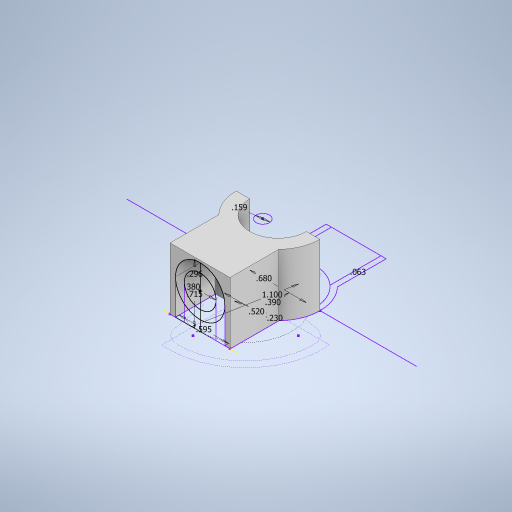
# Autodesk Inventor part: Ball Valve Mount
Saved by Autodesk Inventor 2023 (Build 270158000, 158)
## iProperties
Created: 2023-02-08
Part Number: Ball Valve Mount
Material: Generic
Document SubType Name: Modeling
Designer: tommy
Density: 1 g/cm^3
Appearance: Default
Author: tommy
Autodesk Inventor part; units mm, degrees
ref_plane "YZ Plane" through (0, 0, 0) normal (1, 0, 0) x (0, 1, 0)
ref_plane "XZ Plane" through (0, 0, 0) normal (0, 1, 0) x (-1, 0, 0)
ref_plane "XY Plane" through (0, 0, 0) normal (0, 0, 1) x (1, 0, 0)
sketch "Sketch1" plane through (0, 0, 0) normal (0, 1, 0) x (-1, 0, 0)
  circle A0 centre (0, 0) radius 8.636
  line L0 (7.5565, 23.7871) -> (-7.5565, 23.7871)
  line L1 (7.5565, -23.7871) -> (-7.5565, -23.7871)
  line L2 (7.5565, 23.7871) -> (7.5565, 8.2342)
  line L3 (7.5565, -8.2342) -> (7.5565, -23.7871)
  arc A1 (7.5565, -8.2342) -> (7.5565, 8.2342) centre (0, 0) ccw
  arc A2 (-7.5565, 8.2342) -> (-7.5565, -8.2342) centre (0, 0) ccw
  line L4 (-7.5565, -23.7871) -> (-7.5565, -8.2342)
  line L5 (-7.5565, 8.2342) -> (-7.5565, 23.7871)
  line L6 (-9.144, -8.9047) -> (-9.144, -23.7871)
  line L7 (9.144, -23.7871) -> (9.144, -8.9047)
  arc A3 (9.144, -8.9047) -> (9.144, 8.9047) centre (0, 0) ccw
  line L8 (9.144, 8.9047) -> (9.144, 23.7871)
  line L9 (-9.144, 23.7871) -> (-9.144, 8.9047)
  arc A4 (-9.144, 8.9047) -> (-9.144, -8.9047) centre (0, 0) ccw
  line L10 (7.5565, -23.7871) -> (9.144, -23.7871)
  line L11 (9.144, -23.7871) -> (-9.144, -23.7871)
  line L12 (-7.5565, 23.7871) -> (-9.144, 23.7871)
  line L13 (-9.144, 23.7871) -> (9.144, 23.7871)
  circle A5 centre (0, 0) radius 11.176
  line L14 (46.1577, 0) -> (-42.2099, 0)
  circle A6 centre (20.2123, -15.5184) radius 2.0193
  circle A7 centre (0, 9.906) radius 2.921 construction
  circle A8 centre (0, 9.906) radius 6.604 construction
  line L15 (-6.3706, 3.5354) -> (-16.823, 5.2035) construction
  arc A9 (2.286, 33.1684) -> (-23.2624, 7.62) centre (0, 9.906) ccw construction
  line L16 (4.7025, 26.729) -> (6.3706, 16.2766) construction
  arc A10 (-20.8345, 9.906) -> (-16.823, 5.2035) centre (-16.0725, 9.906) ccw construction
  line L17 (-4.7025, -6.917) -> (-6.3706, 3.5354) construction
  arc A11 (-4.7025, -6.917) -> (0, -10.9285) centre (0, -6.1665) ccw construction
  arc A12 (4.7025, 26.729) -> (0, 30.7405) centre (0, 25.9785) ccw construction
  line L18 (6.3706, 16.2766) -> (16.823, 14.6085) construction
  arc A13 (20.8345, 9.906) -> (16.823, 14.6085) centre (16.0725, 9.906) ccw construction
  arc A14 (0, 30.7405) -> (-20.8345, 9.906) centre (0, 9.906) ccw construction
  arc A15 (0, -10.9285) -> (20.8345, 9.906) centre (0, 9.906) ccw construction
  line L19 (0, 0) -> (0, 9.906)
  line L20 (2.286, 33.2805) -> (2.286, 7.62) construction
  line L21 (2.286, 7.62) -> (-23.3745, 7.62) construction
  circle A16 centre (0, 9.906) radius 13.97 construction
  point P0 (-7.5565, -8.2342)
  point P1 (-7.5565, 8.2342)
  point P2 (-12.7635, 0)
  point P3 (-8.636, 0)
  point P4 (8.636, 0)
  point P5 (12.7635, 0)
  point P6 (-12.7635, 0)
  dimension "d0" = 17.272
  dimension "d6" = 15.113
  dimension "d7" = 1.5875
  dimension "d27" = 4.0386
  dimension "d31" = 5.842
  dimension "d32" = 13.208
  dimension "d35" = 9.906
  dimension "d37" = 27.94
  constraints: 44 end point, 23 point on circle, 17 centre point, 5 coincident, 5 perpendicular, 5 point on line, 3 vertical, 2 horizontal, 1 concentric
  measures "d0" diameter of A0
  measures "d6" distance of L0.start L0.end
  measures "d7" distance between parallel lines of L4 L6
  measures "d27" diameter of A6
  measures "d31" diameter of A7
  measures "d32" diameter of A8
  measures "d35" distance of L19.start L19.end
  measures "d37" diameter of A16
extrude "Extrusion1" add sketch "Sketch1" along normal blind 18.796 contours A0 L14 A2 A5 A1 | A1 L2 L13 L8 A3 L14 | L14 A4 L9 L12 L5 A2 | A5 L5 L0 L2 picked at (-1.5532, 10.1436)
extrude "Extrusion2" cut sketch "Sketch1" along normal blind 2.286 contours L14 A1 A5 A2 A0 | A0 L14 A2 A5 A1
sketch "Sketch2" plane through (-9.144, 0, 23.7871) normal (0, 0, 1) x (1, 0, 0)
  line L0 (9.144, 0) -> (9.144, 18.161)
  line L1 (9.144, 18.161) -> (9.144, 10.6426)
  circle A0 centre (9.144, 10.6426) radius 7.5184
  line L2 (16.6624, 10.6426) -> (16.6624, 0)
  line L3 (20.32, 0) -> (-2.032, 0) projected
  line L4 (1.6256, 10.6426) -> (1.6256, 0)
  line L5 (1.6256, 0) -> (16.6624, 0)
  circle A1 centre (9.144, 10.6426) radius 4.826
  line L6 (4.318, 10.6426) -> (4.318, 0)
  line L7 (13.97, 10.6426) -> (13.97, 0)
  line L8 (18.288, 0) -> (0, 0) projected
  dimension "d12" = 18.161
  dimension "d13" = 7.5184
  dimension "d17" = 9.652
  constraints: 14 end point, 5 point on circle, 5 point on line, 3 perpendicular, 2 centre point, 2 coincident, 2 vertical, 1 parallel
  measures "d12" distance of L0.start L0.end
  measures "d13" distance of L0.end L1.end
  measures "d17" diameter of A1
extrude "Extrusion3" cut sketch "Sketch2" against normal blind 254 contours L3 L6 A0 L0 | L0 A0 L7 L3 | A0 L6 A1 L0 | L0 A1 L7 A0 | A1 L0 | L0 A1 picked at (8.209, 4.1293) picked at (10.079, 4.1293)
extrude "Extrusion4" cut sketch "Sketch2" against normal blind 12.2174 contours L7 A0 L2 L3 | L3 L4 A0 L6 | A0 L0 A1 L6 | L7 A1 L0 A0 picked at (3.9398, 7.1935) picked at (14.3482, 7.1935)
body "Solid1"
